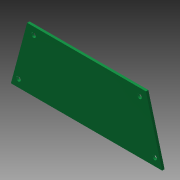
# Autodesk Inventor part: Platine_led
Saved by Autodesk Inventor 2015 (Build 190159000, 159)
## iProperties
Created: 2018-03-07
Part Number: Platine_led
Material: Generisch
Document SubType Name: Modeling
Designer: wepet
Density: 1 g/cm^3
Appearance: Vorgabe
Author: wepet
Autodesk Inventor part; units mm, degrees
ref_plane "YZ Plane" through (0, 0, 0) normal (1, 0, 0) x (0, 1, 0)
ref_plane "XZ Plane" through (0, 0, 0) normal (0, 1, 0) x (-1, 0, 0)
ref_plane "XY Plane" through (0, 0, 0) normal (0, 0, 1) x (1, 0, 0)
sketch "Skizze1" plane through (0, 0, 0) normal (0, 1, 0) x (-1, 0, 0)
  line L0 (50, -20) -> (39.282, 20)
  line L1 (39.282, 20) -> (-39.282, 20)
  line L2 (-39.282, 20) -> (-50, -20)
  line L3 (-50, -20) -> (50, -20)
  line L4 (0, 0) -> (0, -20) construction
  line L5 (0, 0) -> (-44.641, 0) construction
  line L6 (0, 0) -> (0, 20) construction
  line L7 (50, -20) -> (50, 20) construction
  line L8 (50, 20) -> (39.282, 20) construction
  line L9 (45.1166, -15.3499) -> (35, 15) construction
  line L10 (35, 15) -> (-35, 15) construction
  line L11 (-35, 15) -> (-45, -15) construction
  line L12 (-45, -15) -> (45, -15) construction
  circle A0 centre (45, -15) radius 1.5
  circle A1 centre (-45, -15) radius 1.5
  circle A2 centre (-35, 15) radius 1.5
  circle A3 centre (35, 15) radius 1.5
  point P0 (0, -15)
  point P1 (0, 15)
  point P2 (-40, 0)
  dimension "d10" = 100
  dimension "d12" = 40
  dimension "d14" = 15
  dimension "d15" = 90
  dimension "d16" = 70
  dimension "d17" = 30
  dimension "d18" = 3
  dimension "d19" = 3
  dimension "d20" = 3
  dimension "d21" = 3
  constraints: 26 end point, 6 midpoint, 4 centre point, 4 coincident, 4 point on line, 3 vertical, 2 horizontal, 2 perpendicular
  measures "d10" distance of L2.end L0.start
  measures "d12" distance between parallel lines of L1 L3
  measures "d14" angle of L7 L0
  measures "d15" distance of L11.end L12.end
  measures "d16" distance of L9.end L10.end
  measures "d17" distance between parallel lines of L10 L12
  measures "d18" diameter of A0
  measures "d19" diameter of A1
  measures "d20" diameter of A2
  measures "d21" diameter of A3
extrude "Extrusion2" add sketch "Skizze1" along normal blind 1.6
sketch "Skizze2" plane through (0, 1.6, 0) normal (0, 1, 0) x (1, 0, 0)
  circle A0 centre (-35, -15) radius 1.5 construction
  circle A1 centre (35, -15) radius 1.5 construction
  circle A2 centre (45, 15) radius 1.5 construction
  circle A3 centre (-45, 15) radius 1.5 construction
  line L0 (-50, 20) -> (-39.282, -20) construction
  line L1 (-39.282, -20) -> (39.282, -20) construction
  line L2 (39.282, -20) -> (50, 20) construction
  line L3 (50, 20) -> (-50, 20) construction
  line L4 (50, 20) -> (-50, 20) construction
  line L5 (39.282, -20) -> (50, 20) construction
  line L6 (-39.282, -20) -> (39.282, -20) construction
  line L7 (-50, 20) -> (-39.282, -20) construction
  line L8 (-32.5, 0) -> (32.5, 0) construction
  circle A4 centre (-32.5, 0) radius 2.5
  circle A5 centre (32.5, 0) radius 2.5
  point P0 (0, 0)
  point P1 (0, 0)
  dimension "d24" = 65
  dimension "d25" = 5
  dimension "d26" = 5
  constraints: 5 coincident, 2 centre point, 2 end point, 1 horizontal, 1 midpoint
  measures "d24" distance of L8.start L8.end
  measures "d25" diameter of A4
  measures "d26" diameter of A5
extrude "Extrusion3" add sketch "Skizze2" along normal blind 3
